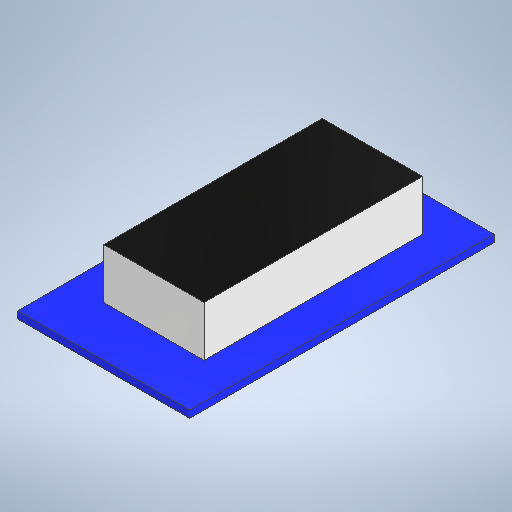
# Autodesk Inventor part: HW-069
Saved by Autodesk Inventor 2025.2 (Build 292293000, 293)
## iProperties
Created: 2026-02-19
Part Number: HW-069
Material: 一般
Document SubType Name: Modeling
Designer: naka6
Density: 1 g/cm^3
Appearance: 既定
Author: naka6
Autodesk Inventor part; units mm, degrees
ref_plane "YZ Plane" through (0, 0, 0) normal (1, 0, 0) x (0, 1, 0)
ref_plane "XZ Plane" through (0, 0, 0) normal (0, 1, 0) x (-1, 0, 0)
ref_plane "XY Plane" through (0, 0, 0) normal (0, 0, 1) x (1, 0, 0)
sketch "スケッチ1" plane through (0, 0, 0) normal (0, 1, 0) x (-1, 0, 0)
  line L0 (12, -21.25) -> (-12, -21.25)
  line L1 (-12, -21.25) -> (-12, 21.25)
  line L2 (-12, 21.25) -> (12, 21.25)
  line L3 (12, 21.25) -> (12, -21.25)
  line L4 (12, -21.25) -> (-12, 21.25) construction
  line L5 (-12, -21.25) -> (12, 21.25) construction
  point P0 (0, 0)
  dimension "d0" = 24
  dimension "d1" = 42.5
  constraints: 12 end point, 2 midpoint, 2 parallel, 1 horizontal, 1 perpendicular
  measures "d0" distance of L1.end L2.end
  measures "d1" distance of L2.end L0.start
extrude "押し出し1" add sketch "スケッチ1" along normal blind 1
sketch "スケッチ2" plane through (0, 0, 0) normal (0, -1, 0) x (1, 0, 0)
  line L0 (-12, 21.25) -> (12, 21.25) projected
  line L1 (-12, -21.25) -> (-12, 21.25) projected
  line L2 (12, -21.25) -> (-12, -21.25) projected
  line L3 (12, 21.25) -> (12, -21.25) projected
  line L4 (-10, 17.25) -> (10, 17.25)
  line L5 (10, 17.25) -> (10, -17.25)
  line L6 (10, -17.25) -> (-10, -17.25)
  line L7 (-10, -17.25) -> (-10, 17.25)
  point P0 (0, 0)
  dimension "d4" = 4
  dimension "d5" = 4
  dimension "d6" = 2
  dimension "d7" = 2
  constraints: 8 end point, 2 parallel, 1 horizontal, 1 perpendicular
  measures "d4" distance between parallel lines of L0 L4
  measures "d5" distance between parallel lines of L2 L6
  measures "d6" distance between parallel lines of L1 L7
  measures "d7" distance between parallel lines of L3 L5
extrude "押し出し2" add sketch "スケッチ2" along normal blind 2 contours L4 L5 L6 L7
sketch "スケッチ3" plane through (0, 1, 0) normal (0, 1, 0) x (1, 0, 0)
  line L0 (7, -14.25) -> (-7, -14.25)
  line L1 (-7, -14.25) -> (-7, 16.25)
  line L2 (-7, 16.25) -> (7, 16.25)
  line L3 (7, 16.25) -> (7, -14.25)
  line L4 (-12, -21.25) -> (12, -21.25) projected
  line L5 (12, 21.25) -> (-12, 21.25) projected
  line L6 (12, -21.25) -> (12, 21.25) projected
  line L7 (-12, 21.25) -> (-12, -21.25) projected
  point P0 (0, 0)
  dimension "d10" = 7
  dimension "d11" = 5
  dimension "d12" = 5
  dimension "d13" = 5
  constraints: 8 end point, 2 parallel, 1 horizontal, 1 perpendicular
  measures "d10" distance between parallel lines of L4 L0
  measures "d11" distance between parallel lines of L2 L5
  measures "d12" distance between parallel lines of L6 L3
  measures "d13" distance between parallel lines of L7 L1
extrude "押し出し3" add sketch "スケッチ3" along normal blind 7 contours L0 L1 L2 L3
